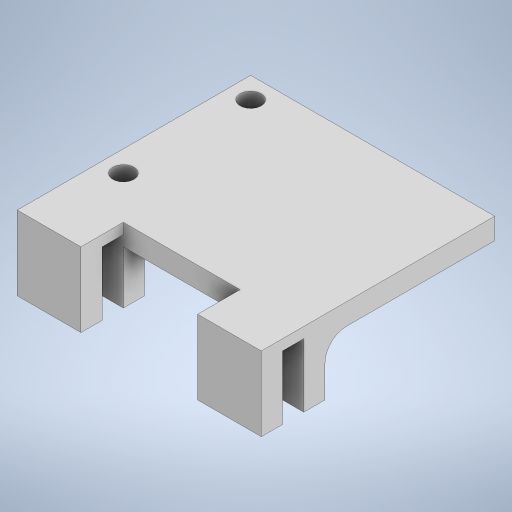
# Autodesk Inventor part: sensor
Saved by Autodesk Inventor 2024 (Build 280153000, 153)
## iProperties
Created: 2024-04-17
Part Number: sensor
Material: Generic
Document SubType Name: Modeling
Designer: 22546723
Density: 1 g/cm^3
Appearance: Default
Author: 22546723
## iProperties of the stored document sensor_3DPrint.ipt
Created: 2024-04-17
Part Number: sensor_3DPrint
Material: Generic
Document SubType Name: Modeling
Designer: 22546723
Density: 1 g/cm^3
Appearance: Default
Author: 22546723
Autodesk Inventor part; units mm, degrees
ref_plane "YZ Plane" through (0, 0, 0) normal (1, 0, 0) x (0, 1, 0)
ref_plane "XZ Plane" through (0, 0, 0) normal (0, 1, 0) x (-1, 0, 0)
ref_plane "XY Plane" through (0, 0, 0) normal (0, 0, 1) x (1, 0, 0)
sketch "Sketch1" plane through (0, 0, 0) normal (0, 1, 0) x (-1, 0, 0)
  line L0 (-5.5, -3) -> (-11.5, -3)
  line L1 (-11.5, -3) -> (-11.5, 3)
  line L2 (-11.5, 3) -> (-5.5, 3)
  line L3 (-5.5, 3) -> (-5.5, -3)
  line L4 (-5.5, -3) -> (-11.5, 3) construction
  line L5 (-11.5, -3) -> (-5.5, 3) construction
  line L6 (11.5, -3) -> (5.5, -3)
  line L7 (5.5, -3) -> (5.5, 3)
  line L8 (5.5, 3) -> (11.5, 3)
  line L9 (11.5, 3) -> (11.5, -3)
  line L10 (11.5, -3) -> (5.5, 3) construction
  line L11 (5.5, -3) -> (11.5, 3) construction
  point P0 (0, 0)
  point P1 (-8.5, 0)
  point P2 (8.5, 0)
  dimension "d0" = 6
  dimension "d1" = 6
  dimension "d2" = 0
  dimension "d3" = 5.5
  dimension "d4" = 6
  dimension "d5" = 6
  dimension "d7" = 11
  constraints: 24 end point, 4 midpoint, 4 parallel, 2 horizontal, 2 perpendicular, 1 collinear
  measures "d0" distance of L1.end L2.end
  measures "d1" distance between parallel lines of L2 L0
  measures "d2" vertical distance of point (-8.5, 0) point (0, 0)
  measures "d3" distance from line of L3 point (0, 0)
  measures "d4" distance of L7.end L8.end
  measures "d5" distance between parallel lines of L8 L6
  measures "d7" distance between parallel lines of L3 L7
extrude "Extrusion1" add sketch "Sketch1" against normal blind 1
sketch "Sketch2" plane through (0, -1, 0) normal (0, -1, 0) x (1, 0, 0)
  line L0 (-5.5, 3) -> (-11.5, 3) projected
  line L1 (-5.5, 3) -> (-5.5, -3) projected
  line L2 (-11.5, 3) -> (-5.5, 3)
  line L3 (-5.5, 3) -> (-5.5, 1)
  line L4 (-5.5, 1) -> (-11.5, 1)
  line L5 (-11.5, 1) -> (-11.5, 3)
  line L6 (-5.5, -3) -> (-11.5, -3) projected
  line L7 (-11.5, -3) -> (-5.5, -3)
  line L8 (-5.5, -3) -> (-5.5, -1)
  line L9 (-5.5, -1) -> (-11.5, -1)
  line L10 (-11.5, -1) -> (-11.5, -3)
  line L11 (5.5, 3) -> (5.5, -3) projected
  line L12 (11.5, -3) -> (11.5, 3) projected
  line L13 (5.5, 3) -> (11.5, 3)
  line L14 (11.5, 3) -> (11.5, 1)
  line L15 (11.5, 1) -> (5.5, 1)
  line L16 (5.5, 1) -> (5.5, 3)
  line L17 (5.5, -3) -> (11.5, -3) projected
  line L18 (5.5, -3) -> (11.5, -3)
  line L19 (11.5, -3) -> (11.5, -1)
  line L20 (11.5, -1) -> (5.5, -1)
  line L21 (5.5, -1) -> (5.5, -3)
  point P0 (0, 0)
  dimension "d10" = 2
  dimension "d11" = 2
  constraints: 32 end point, 8 parallel, 4 horizontal, 4 perpendicular, 4 point on line, 2 collinear
  measures "d10" distance between parallel lines of L0 L4
  measures "d11" distance between parallel lines of L6 L9
extrude "Extrusion2" add sketch "Sketch2" along normal blind 6 contours L1 L4 L5 L0 | L1 L6 L10 L9 | L13 L12 L15 L11 | L20 L12 L17 L11
sketch "Sketch3" plane through (0, 0, 0) normal (0, 1, 0) x (1, 0, 0)
  line L0 (-11.5, 1) -> (-11.5, 3) projected
  line L1 (-11.5, 1) -> (11.5, 1)
  line L2 (11.5, 1) -> (11.5, 19)
  line L3 (11.5, 19) -> (-11.5, 19)
  line L4 (-11.5, 19) -> (-11.5, 1)
  line L5 (-5.5, 3) -> (-11.5, 3) projected
  circle A0 centre (-9.5, 17) radius 1
  circle A1 centre (-9.5, 5) radius 1
  point P0 (0, 0)
  dimension "d14" = 23
  dimension "d15" = 16
  dimension "d16" = 2
  dimension "d17" = 2
  dimension "d18" = 2
  dimension "d19" = 2
  dimension "d20" = 2
  dimension "d21" = 2
  constraints: 8 end point, 2 centre point, 2 parallel, 1 horizontal, 1 perpendicular
  measures "d14" distance of L3.end L2.end
  measures "d15" distance between parallel lines of L5 L3
  measures "d16" diameter of A0
  measures "d17" diameter of A1
  measures "d18" distance from line of L3 A0.centre
  measures "d19" distance from line of L4 A0.centre
  measures "d20" distance from line of L5 A1.centre
  measures "d21" distance from line of L4 A1.centre
extrude "Extrusion3" add sketch "Sketch3" against normal blind 2
fillet "Fillet1" radius 2 2 edges at (-8.5, -2, -3) (8.5, -2, -3)
body "Solid1"
